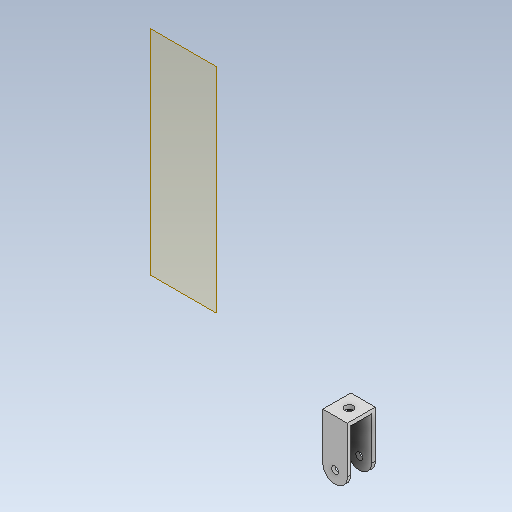
# Autodesk Inventor part: Junta Revoluta
Saved by Autodesk Inventor 2021 (Build 250183000, 183)
## iProperties
Created: 2021-07-14
Part Number: Junta Revoluta
Material: Generic
Document SubType Name: Modeling
Designer: maaro
Density: 1 g/cm^3
Appearance: Default
Author: maaro
Autodesk Inventor part; units mm, degrees
ref_plane "YZ Plane" through (0, 0, 0) normal (1, 0, 0) x (0, 1, 0)
ref_plane "XZ Plane" through (0, 0, 0) normal (0, 1, 0) x (-1, 0, 0)
ref_plane "XY Plane" through (0, 0, 0) normal (0, 0, 1) x (1, 0, 0)
ref_plane "Work Plane1" through (0, 0, 0) normal (0, 0, 1) x (1, 0, 0)
sketch "Sketch1" plane through (0, 0, 0) normal (0, 0, 1) x (1, 0, 0)
  line L0 (55, -528.7123) -> (55, -461.767)
  line L1 (55, -461.767) -> (20, -461.767)
  line L2 (20, -461.767) -> (20, -528.7123)
  arc A0 (20, -528.7123) -> (55, -528.7123) centre (37.5, -528.7123) ccw
  line L3 (43.5, -461.767) -> (31.5, -461.767) projected
  line L4 (37.5, -461.767) -> (37.5, -485.2876) construction
  arc A1 (30.6824, -513.1447) -> (23.108, -519.6737) centre (26.8952, -516.4092) ccw projected
  line L5 (88.3973, -595.4186) -> (23.108, -519.6737) projected
  line L6 (30.6824, -513.1447) -> (95.9718, -588.8897) projected
  arc A2 (88.3973, -595.4186) -> (95.9718, -588.8897) centre (92.1846, -592.1541) ccw projected
  line L7 (92.1846, -592.1541) -> (26.8952, -516.4092) construction
  circle A3 centre (37.5, -528.7123) radius 5
  point P0 (0, 0)
  dimension "d0" = 23.5206
  dimension "d1" = 35
  constraints: 10 end point, 3 tangent, 2 centre point, 2 perpendicular, 2 point on circle, 2 point on line, 2 vertical, 1 coincident, 1 collinear, 1 midpoint
  measures "d0" distance of L4.start L4.end
  measures "d1" distance of L0.end L1.end
extrude "Extrusion1" add sketch "Sketch1" along normal mid plane 40 contours A0 L6 A1 L5 L2 L1 L0 | A0 L5 A3 L6 | A3 L5 A1 L6
sketch "Sketch2" plane through (20, -528.7123, 20) normal (-1, 0, 0) x (0, 0, 1)
  line L0 (-11, 54.2123) -> (-29, 54.2123) projected
  line L1 (-11, 61.2123) -> (-29, 61.2123) projected
  line L2 (-34.8412, -128.9954) -> (-34.8412, 22.4945) projected
  line L3 (-4.8412, 22.4945) -> (-4.8412, -128.9954) projected
  line L4 (-40, -17.5) -> (0, -17.5) projected
  line L5 (-4.8412, -17.5) -> (-4.8412, 61.2123)
  line L6 (-4.8412, 61.2123) -> (-34.8412, 61.2123)
  line L7 (-34.8412, 61.2123) -> (-34.8412, -17.5)
  point P0 (-20, 528.7123)
  point P1 (-34.8412, 22.4945)
  point P2 (-29, 61.2123)
  constraints: 6 end point, 5 point on line, 1 collinear, 1 perpendicular, 1 vertical
extrude "Extrusion2" cut sketch "Sketch2" against normal through all
sketch "Sketch3" plane through (20, -467.5, -14.8412) normal (0, -1, 0) x (1, 0, 0)
  circle A0 centre (17.5, 14.8412) radius 6 projected
  point P0 (-20, 14.8412)
extrude "Extrusion3" cut sketch "Sketch3" against normal through all
body "Solid1"
